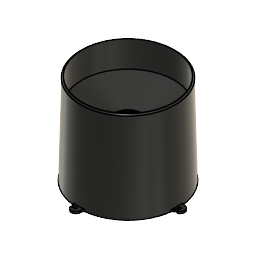
Top Component (FA1) (Autodesk Fusion 360 design; units mm, degrees)
Autodesk Fusion 360 part; units mm, degrees
sketch "Sketch1" plane through (0, 0, 0) normal (0, 0, 1) x (1, 0, 0)
  circle A0 centre (0, 0) radius 110
  circle A1 centre (0, 0) radius 106.5
  arc A2 (10.2564, 113.75) -> (12.5979, 109.2762) centre (20, 116) ccw
  arc A3 (9.7436, 118.25) -> (-10, 116) centre (0, 116) ccw
  arc A4 (-12.5979, 109.2762) -> (-10, 116) centre (-20, 116) ccw
  line L0 (0, 113.75) -> (10.2564, 113.75)
  line L1 (9.7436, 118.25) -> (0, 118.25)
  arc A5 (0, 118.25) -> (0, 113.75) centre (0, 116) ccw
  line L2 (12.5979, 109.2762) -> (12.5979, 107)
  line L3 (12.5979, 107) -> (-12.5979, 107)
  line L4 (-12.5979, 107) -> (-12.5979, 109.2762)
  dimension "d1" = 220
  dimension "d2" = 213
  dimension "d41" = 4.5
  dimension "d54" = 7.75
  dimension "d55" = 12.5979
  dimension "d56" = 107
  dimension "d57" = 11.25
  dimension "d58" = 40
  dimension "d59" = 10.2564
  constraint coincident A0.centre A1.centre
  constraint concentric A0 A1
  constraint parallel L0 L1
  constraint vertical L2
  constraint perpendicular L2 L3
  constraint perpendicular L3 L4
  constraint tangent L0 A5
  constraint tangent L1 A5
  constraint concentric A3 A5
  constraint coincident A0 A2.end
  constraint vertical A0.centre L0.start
  constraint equal A2 A3
  constraint equal A2 A4
  constraint coincident A3.end A4.end
  constraint parallel L0 L3
  constraint equal L2 L4
  measures "d1" diameter of A0
  measures "d2" diameter of A1
  measures "d41" diameter of A5
  measures "d54" distance of A3 A5
  measures "d55" distance of A0.centre L4
  measures "d56" distance of A0.centre L3
  measures "d57" distance of A3.start L3
  measures "d58" horizontal distance of A4.centre A2.centre
  measures "d59" distance of L0.start A2.start
ref_plane "WorkPlane1" through (0, 0, 220) normal (0, 0, 1) x (1, 0, 0)
sketch "Sketch2" plane through (0, 0, 220) normal (0, 0, 1) x (1, 0, 0)
  circle A0 centre (0, 0) radius 105
  circle A1 centre (0, 0) radius 101.5
  dimension "d4" = 210
  dimension "d5" = 203
  constraint coincident A0.centre A1.centre
  measures "d4" diameter of A0
  measures "d5" diameter of A1
sketch "Sketch3" plane through (0, 0, 0) normal (0, 1, 0) x (1, 0, 0)
  line L0 (0, 0) -> (-110, 0) construction
  line L1 (-110, 0) -> (-106.5, 0)
  line L2 (0, -200) -> (-105, -200) construction
  line L3 (-105, -200) -> (-101.5, -200)
  line L4 (-105, -200) -> (-110, 0)
  line L5 (-106.5, 0) -> (-101.5, -200)
  line L6 (0, 0) -> (0, -10) construction
  line L7 (0, -10) -> (0, -200) construction
  dimension "d6" = 110
  dimension "d7" = 3.5
  dimension "d8" = 105
  dimension "d9" = 3.5
  dimension "d42" = 190
  dimension "d60" = 200
  constraint coincident L0.start L6.start
  constraint horizontal L0
  constraint parallel L0 L1
  constraint horizontal L2
  constraint parallel L2 L3
  constraint perpendicular L0 L6
  constraint perpendicular L0 L7
  constraint coincident L2.start L7.end
  measures "d6" distance of L0.start L0.end
  measures "d7" distance of L0.end L1.end
  measures "d8" distance of L2.start L2.end
  measures "d9" distance of L2.end L3.end
  measures "d42" distance of L6.end L2.start
  measures "d60" distance of L0 L2
revolve "Revolve1" add sketch "Sketch3" angle 360 about axis through (0, 0, 1.75) along (0, 0, 1) makes body 1
extrude "Extrude1" add sketch "Sketch1" along normal blind 4 contours A0 L2 L3 L4 | A0 A2 A3 A4 L0 L1 A5 picked at (1.4025, 107.9732) bodies 1
pattern_circular "C-Pattern1" count 4 over 360 about axis through (0, 0, 1.75) along (0, 0, 1) of "Extrude1"
ref_plane "WorkPlane2" through (0, 0, 110) normal (0, 0, 1) x (1, 0, 0)
sketch "Sketch5" plane through (0, 0, 0) normal (0, 1, 0) x (-1, 0, 0)
  line L0 (-30, 114) -> (-103.6332, 140.8003)
  line L1 (-0.0018, 113.6676) -> (57.7728, 113.6676) construction
  line L2 (-103.6332, 140.8003) -> (-106.3694, 133.2828)
  line L3 (-106.3694, 133.2828) -> (-31.4106, 106)
  line L4 (-30, 114) -> (-30, 106)
  line L5 (-30, 106) -> (-31.4106, 106)
  line L6 (0, 0) -> (0, 110) construction
  point P0 (-30, 110)
  dimension "d47" = 30
  dimension "d49" = 160
  dimension "d50" = 8
  dimension "d51" = 8
  dimension "d52" = 110
  dimension "d61" = 0.3324
  dimension "d62" = 34.8003
  dimension "d63" = 57.7746
  constraint horizontal L1
  constraint perpendicular L0 L2
  constraint parallel L0 L3
  constraint perpendicular L4 L5
  constraint coincident L6.start origin
  constraint perpendicular L1 L6
  constraint midpoint L4 P0
  constraint vertical L4.end P0
  measures "d47" distance of L1.start L0.start
  measures "d49" angle of L0 L1
  measures "d50" distance of L0.end L2.end
  measures "d51" distance of L0.start L4.end
  measures "d52" distance of L6.start L6.end
  measures "d61" distance of L0.start L1
  measures "d62" vertical distance of L0.end L3.end
  measures "d63" horizontal distance of L1.start L1.end
sketch "Sketch4" plane through (0, 0, 110) normal (0, 0, 1) x (1, 0, 0)
  circle A0 centre (0, 0) radius 105.125
  circle A1 centre (0, 0) radius 30
  line L0 (2.5, 2.5) -> (-2.5, 2.5)
  line L1 (-2.5, 2.5) -> (-2.5, -2.5)
  line L2 (-2.5, -2.5) -> (2.5, -2.5)
  line L3 (2.5, -2.5) -> (2.5, 2.5)
  line L4 (2.5, 2.5) -> (-2.5, -2.5) construction
  line L5 (-2.5, 2.5) -> (2.5, -2.5) construction
  line L6 (-10, -27.5) -> (-10, -28.2843)
  line L7 (-5, -27.5) -> (-10, -27.5)
  line L8 (-5, -29.5804) -> (-5, -27.5)
  line L9 (-2.5, -27.5) -> (-2.5, -29.8957)
  line L10 (2.5, -27.5) -> (-2.5, -27.5)
  line L11 (2.5, -29.8957) -> (2.5, -27.5)
  line L12 (5, -27.5) -> (5, -29.5804)
  line L13 (10, -27.5) -> (5, -27.5)
  line L14 (10, -28.2843) -> (10, -27.5)
  line L15 (-20, -20) -> (-22.3607, -20)
  line L16 (-20, -22.3607) -> (-20, -20)
  line L17 (-17.5, -20) -> (-17.5, -24.367)
  line L18 (-16.5831, -25) -> (-12.5, -25)
  line L19 (-12.5, -20) -> (-17.5, -20)
  line L20 (-12.5, -25) -> (-12.5, -20)
  line L21 (-10, -20) -> (-10, -25)
  line L22 (-10, -25) -> (-5, -25)
  line L23 (-5, -20) -> (-10, -20)
  line L24 (-5, -25) -> (-5, -20)
  line L25 (-2.5, -20) -> (-2.5, -25)
  line L26 (-2.5, -25) -> (2.5, -25)
  line L27 (2.5, -20) -> (-2.5, -20)
  line L28 (2.5, -25) -> (2.5, -20)
  line L29 (5, -20) -> (5, -25)
  line L30 (5, -25) -> (10, -25)
  line L31 (10, -20) -> (5, -20)
  line L32 (10, -25) -> (10, -20)
  line L33 (12.5, -20) -> (12.5, -25)
  line L34 (12.5, -25) -> (16.5831, -25)
  line L35 (17.5, -20) -> (12.5, -20)
  line L36 (17.5, -24.367) -> (17.5, -20)
  line L37 (20, -20) -> (20, -22.3607)
  line L38 (22.3607, -20) -> (20, -20)
  line L39 (-25, -12.5) -> (-25, -16.5831)
  line L40 (-24.367, -17.5) -> (-20, -17.5)
  line L41 (-20, -12.5) -> (-25, -12.5)
  line L42 (-20, -17.5) -> (-20, -12.5)
  line L43 (-17.5, -12.5) -> (-17.5, -17.5)
  line L44 (-17.5, -17.5) -> (-12.5, -17.5)
  line L45 (-12.5, -12.5) -> (-17.5, -12.5)
  line L46 (-12.5, -17.5) -> (-12.5, -12.5)
  line L47 (-10, -12.5) -> (-10, -17.5)
  line L48 (-10, -17.5) -> (-5, -17.5)
  line L49 (-5, -12.5) -> (-10, -12.5)
  line L50 (-5, -17.5) -> (-5, -12.5)
  line L51 (-2.5, -12.5) -> (-2.5, -17.5)
  line L52 (-2.5, -17.5) -> (2.5, -17.5)
  line L53 (2.5, -12.5) -> (-2.5, -12.5)
  line L54 (2.5, -17.5) -> (2.5, -12.5)
  line L55 (5, -12.5) -> (5, -17.5)
  line L56 (5, -17.5) -> (10, -17.5)
  line L57 (10, -12.5) -> (5, -12.5)
  line L58 (10, -17.5) -> (10, -12.5)
  line L59 (12.5, -12.5) -> (12.5, -17.5)
  line L60 (12.5, -17.5) -> (17.5, -17.5)
  line L61 (17.5, -12.5) -> (12.5, -12.5)
  line L62 (17.5, -17.5) -> (17.5, -12.5)
  line L63 (20, -12.5) -> (20, -17.5)
  line L64 (20, -17.5) -> (24.367, -17.5)
  line L65 (25, -12.5) -> (20, -12.5)
  line L66 (25, -16.5831) -> (25, -12.5)
  line L67 (-28.2843, -10) -> (-27.5, -10)
  line L68 (-27.5, -5) -> (-29.5804, -5)
  line L69 (-27.5, -10) -> (-27.5, -5)
  line L70 (-25, -5) -> (-25, -10)
  line L71 (-25, -10) -> (-20, -10)
  line L72 (-20, -5) -> (-25, -5)
  line L73 (-20, -10) -> (-20, -5)
  line L74 (-17.5, -5) -> (-17.5, -10)
  line L75 (-17.5, -10) -> (-12.5, -10)
  line L76 (-12.5, -5) -> (-17.5, -5)
  line L77 (-12.5, -10) -> (-12.5, -5)
  line L78 (-10, -5) -> (-10, -10)
  line L79 (-10, -10) -> (-5, -10)
  line L80 (-5, -5) -> (-10, -5)
  line L81 (-5, -10) -> (-5, -5)
  line L82 (-2.5, -5) -> (-2.5, -10)
  line L83 (-2.5, -10) -> (2.5, -10)
  line L84 (2.5, -5) -> (-2.5, -5)
  line L85 (2.5, -10) -> (2.5, -5)
  line L86 (5, -5) -> (5, -10)
  line L87 (5, -10) -> (10, -10)
  line L88 (10, -5) -> (5, -5)
  line L89 (10, -10) -> (10, -5)
  line L90 (12.5, -5) -> (12.5, -10)
  line L91 (12.5, -10) -> (17.5, -10)
  line L92 (17.5, -5) -> (12.5, -5)
  line L93 (17.5, -10) -> (17.5, -5)
  line L94 (20, -5) -> (20, -10)
  line L95 (20, -10) -> (25, -10)
  line L96 (25, -5) -> (20, -5)
  line L97 (25, -10) -> (25, -5)
  line L98 (27.5, -5) -> (27.5, -10)
  line L99 (27.5, -10) -> (28.2843, -10)
  line L100 (29.5804, -5) -> (27.5, -5)
  line L101 (-29.8957, -2.5) -> (-27.5, -2.5)
  line L102 (-27.5, 2.5) -> (-29.8957, 2.5)
  line L103 (-27.5, -2.5) -> (-27.5, 2.5)
  line L104 (-25, 2.5) -> (-25, -2.5)
  line L105 (-25, -2.5) -> (-20, -2.5)
  line L106 (-20, 2.5) -> (-25, 2.5)
  line L107 (-20, -2.5) -> (-20, 2.5)
  line L108 (-17.5, 2.5) -> (-17.5, -2.5)
  line L109 (-17.5, -2.5) -> (-12.5, -2.5)
  line L110 (-12.5, 2.5) -> (-17.5, 2.5)
  line L111 (-12.5, -2.5) -> (-12.5, 2.5)
  line L112 (-10, 2.5) -> (-10, -2.5)
  line L113 (-10, -2.5) -> (-5, -2.5)
  line L114 (-5, 2.5) -> (-10, 2.5)
  line L115 (-5, -2.5) -> (-5, 2.5)
  line L116 (5, 2.5) -> (5, -2.5)
  line L117 (5, -2.5) -> (10, -2.5)
  line L118 (10, 2.5) -> (5, 2.5)
  line L119 (10, -2.5) -> (10, 2.5)
  line L120 (12.5, 2.5) -> (12.5, -2.5)
  line L121 (12.5, -2.5) -> (17.5, -2.5)
  line L122 (17.5, 2.5) -> (12.5, 2.5)
  line L123 (17.5, -2.5) -> (17.5, 2.5)
  line L124 (20, 2.5) -> (20, -2.5)
  line L125 (20, -2.5) -> (25, -2.5)
  line L126 (25, 2.5) -> (20, 2.5)
  line L127 (25, -2.5) -> (25, 2.5)
  line L128 (27.5, 2.5) -> (27.5, -2.5)
  line L129 (27.5, -2.5) -> (29.8957, -2.5)
  line L130 (29.8957, 2.5) -> (27.5, 2.5)
  line L131 (-29.5804, 5) -> (-27.5, 5)
  line L132 (-27.5, 10) -> (-28.2843, 10)
  line L133 (-27.5, 5) -> (-27.5, 10)
  line L134 (-25, 10) -> (-25, 5)
  line L135 (-25, 5) -> (-20, 5)
  line L136 (-20, 10) -> (-25, 10)
  line L137 (-20, 5) -> (-20, 10)
  line L138 (-17.5, 10) -> (-17.5, 5)
  line L139 (-17.5, 5) -> (-12.5, 5)
  line L140 (-12.5, 10) -> (-17.5, 10)
  line L141 (-12.5, 5) -> (-12.5, 10)
  line L142 (-10, 10) -> (-10, 5)
  line L143 (-10, 5) -> (-5, 5)
  line L144 (-5, 10) -> (-10, 10)
  line L145 (-5, 5) -> (-5, 10)
  line L146 (-2.5, 10) -> (-2.5, 5)
  line L147 (-2.5, 5) -> (2.5, 5)
  line L148 (2.5, 10) -> (-2.5, 10)
  line L149 (2.5, 5) -> (2.5, 10)
  line L150 (5, 10) -> (5, 5)
  line L151 (5, 5) -> (10, 5)
  line L152 (10, 10) -> (5, 10)
  line L153 (10, 5) -> (10, 10)
  line L154 (12.5, 10) -> (12.5, 5)
  line L155 (12.5, 5) -> (17.5, 5)
  line L156 (17.5, 10) -> (12.5, 10)
  line L157 (17.5, 5) -> (17.5, 10)
  line L158 (20, 10) -> (20, 5)
  line L159 (20, 5) -> (25, 5)
  line L160 (25, 10) -> (20, 10)
  line L161 (25, 5) -> (25, 10)
  line L162 (27.5, 10) -> (27.5, 5)
  line L163 (27.5, 5) -> (29.5804, 5)
  line L164 (28.2843, 10) -> (27.5, 10)
  line L165 (-25, 16.5831) -> (-25, 12.5)
  line L166 (-25, 12.5) -> (-20, 12.5)
  line L167 (-20, 17.5) -> (-24.367, 17.5)
  line L168 (-20, 12.5) -> (-20, 17.5)
  line L169 (-17.5, 17.5) -> (-17.5, 12.5)
  line L170 (-17.5, 12.5) -> (-12.5, 12.5)
  line L171 (-12.5, 17.5) -> (-17.5, 17.5)
  line L172 (-12.5, 12.5) -> (-12.5, 17.5)
  line L173 (-10, 17.5) -> (-10, 12.5)
  line L174 (-10, 12.5) -> (-5, 12.5)
  line L175 (-5, 17.5) -> (-10, 17.5)
  line L176 (-5, 12.5) -> (-5, 17.5)
  line L177 (-2.5, 17.5) -> (-2.5, 12.5)
  line L178 (-2.5, 12.5) -> (2.5, 12.5)
  line L179 (2.5, 17.5) -> (-2.5, 17.5)
  line L180 (2.5, 12.5) -> (2.5, 17.5)
  line L181 (5, 17.5) -> (5, 12.5)
  line L182 (5, 12.5) -> (10, 12.5)
  line L183 (10, 17.5) -> (5, 17.5)
  line L184 (10, 12.5) -> (10, 17.5)
  line L185 (12.5, 17.5) -> (12.5, 12.5)
  line L186 (12.5, 12.5) -> (17.5, 12.5)
  line L187 (17.5, 17.5) -> (12.5, 17.5)
  line L188 (17.5, 12.5) -> (17.5, 17.5)
  line L189 (20, 17.5) -> (20, 12.5)
  line L190 (20, 12.5) -> (25, 12.5)
  line L191 (24.367, 17.5) -> (20, 17.5)
  line L192 (25, 12.5) -> (25, 16.5831)
  line L193 (-22.3607, 20) -> (-20, 20)
  line L194 (-20, 20) -> (-20, 22.3607)
  line L195 (-17.5, 24.367) -> (-17.5, 20)
  line L196 (-17.5, 20) -> (-12.5, 20)
  line L197 (-12.5, 25) -> (-16.5831, 25)
  line L198 (-12.5, 20) -> (-12.5, 25)
  line L199 (-10, 25) -> (-10, 20)
  line L200 (-10, 20) -> (-5, 20)
  line L201 (-5, 25) -> (-10, 25)
  line L202 (-5, 20) -> (-5, 25)
  line L203 (-2.5, 25) -> (-2.5, 20)
  line L204 (-2.5, 20) -> (2.5, 20)
  line L205 (2.5, 25) -> (-2.5, 25)
  line L206 (2.5, 20) -> (2.5, 25)
  line L207 (5, 25) -> (5, 20)
  line L208 (5, 20) -> (10, 20)
  line L209 (10, 25) -> (5, 25)
  line L210 (10, 20) -> (10, 25)
  line L211 (12.5, 25) -> (12.5, 20)
  line L212 (12.5, 20) -> (17.5, 20)
  line L213 (16.5831, 25) -> (12.5, 25)
  line L214 (17.5, 20) -> (17.5, 24.367)
  line L215 (20, 22.3607) -> (20, 20)
  line L216 (20, 20) -> (22.3607, 20)
  line L217 (-10, 28.2843) -> (-10, 27.5)
  line L218 (-10, 27.5) -> (-5, 27.5)
  line L219 (-5, 27.5) -> (-5, 29.5804)
  line L220 (-2.5, 29.8957) -> (-2.5, 27.5)
  line L221 (-2.5, 27.5) -> (2.5, 27.5)
  line L222 (2.5, 27.5) -> (2.5, 29.8957)
  line L223 (5, 29.5804) -> (5, 27.5)
  line L224 (5, 27.5) -> (10, 27.5)
  line L225 (10, 27.5) -> (10, 28.2843)
  dimension "d27" = 210.25
  dimension "d28" = 60
  dimension "d29" = 5
  dimension "d30" = 5
  constraint coincident A0.centre A1.centre
  constraint concentric A0 A1
  constraint horizontal L0
  constraint perpendicular L0 L1
  constraint parallel L0 L2
  constraint parallel L1 L3
  constraint coincident L4 A0.centre
  constraint coincident L5 A0.centre
  constraint coincident A1 L217.start
  constraint coincident A1 L219.end
  constraint coincident A1 L220.start
  constraint coincident A1 L222.end
  constraint coincident A1 L223.start
  constraint coincident A1 L225.end
  constraint coincident A1 L194.end
  constraint coincident A1 L193.start
  constraint coincident A1 L167.end
  constraint coincident A1 L165.start
  constraint coincident A1 L197.end
  constraint coincident A1 L195.start
  constraint coincident A1 L132.end
  constraint coincident A1 L131.start
  constraint coincident A1 L102.end
  constraint coincident A1 L101.start
  constraint coincident A1 L68.end
  constraint coincident A1 L67.start
  constraint coincident A1 L39.end
  constraint coincident A1 L40.start
  constraint coincident A1 L15.end
  constraint coincident A1 L16.start
  constraint coincident A1 L17.end
  constraint coincident A1 L18.start
  constraint coincident A1 L6.end
  constraint coincident A1 L8.start
  constraint coincident A1 L9.end
  constraint coincident A1 L11.start
  constraint coincident A1 L12.end
  constraint coincident A1 L14.start
  constraint coincident A1 L34.end
  constraint coincident A1 L36.start
  constraint coincident A1 L37.end
  constraint coincident A1 L38.start
  constraint coincident A1 L66.start
  constraint coincident A1 L64.end
  constraint coincident A1 L100.start
  constraint coincident A1 L99.end
  constraint coincident A1 L130.start
  constraint coincident A1 L129.end
  constraint coincident A1 L163.end
  constraint coincident A1 L164.start
  constraint coincident A1 L191.start
  constraint coincident A1 L192.end
  constraint coincident A1 L216.end
  constraint coincident A1 L215.start
  constraint coincident A1 L213.start
  constraint coincident A1 L214.end
  measures "d27" diameter of A0
  measures "d28" diameter of A1
  measures "d29" distance of L1.end L2.end
  measures "d30" distance of L0.end L1.end
extrude "Extrude2" add sketch "Sketch4" along normal mid plane 8 separate body contours A1 L6 L7 L8 L9 L10 L11 L12 L13 L14 L15 L16 L17 L18 L19 L20 L33 L34 L35 L36 L37 L38 L39 L40 L41 L42 L63 L64 L65 L66 L67 L68 L69 L98 L99 L100 L101 L102 L103 L128 L129 L130 L131 L132 L133 L162 L163 L164 L165 L166 L167 L168 L189 L190 L191 L192 L193 L194 L195 L196 L197 L198 L211 L212 L213 L214 L215 L216 L217 L218 L219 L220 L221 L222 L223 L224 L225 makes body 2
revolve "Revolve2" add sketch "Sketch5" angle 360 about axis through (0, 0, 0) along (0, 0, 1) bodies 1 2
chamfer "Chamfer1" distance 3 angle 45 1 edges at (-97.8944, 37.9696, 200) on bodies 1
equation "d8 = ( 210 / 2 ) * 1 mm"
equation "d27 = ( ( ( 220 - 5 ) + ( 210.5 - 5 ) ) / 2 ) * 1 mm"
